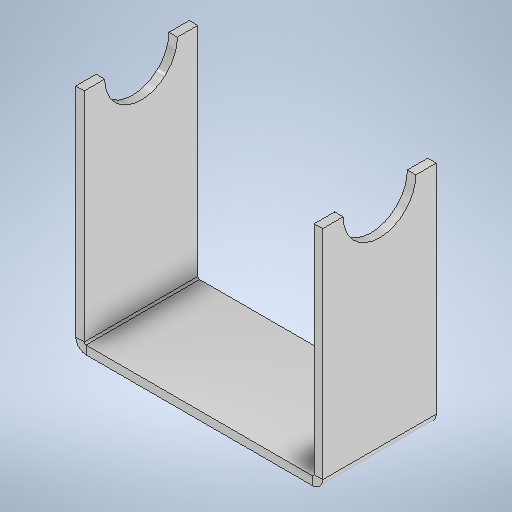
# Autodesk Inventor part: axis_10_top_frame
Saved by Autodesk Inventor 2025.2 (Build 292293000, 293)
## iProperties
Created: 2025-05-04
Part Number: axis_10_top_frame
Material: Aluminum 6061-AHC
Document SubType Name: Sheet Metal
Designer: User
Density: 2.7 g/cm^3
Sheet Metal Rule: Default_mm
Appearance: Aluminum - Dark
Author: User
Autodesk Inventor part; units mm, degrees
ref_plane "YZ Plane" through (0, 0, 0) normal (1, 0, 0) x (0, 1, 0)
ref_plane "XZ Plane" through (0, 0, 0) normal (0, 1, 0) x (-1, 0, 0)
ref_plane "XY Plane" through (0, 0, 0) normal (0, 0, 1) x (1, 0, 0)
sketch "Sketch1" plane through (0, 0, 0) normal (0, 1, 0) x (-1, 0, 0)
  line L0 (20.25, -10) -> (-20.25, -10)
  line L1 (-20.25, -10) -> (-20.25, 10)
  line L2 (-20.25, 10) -> (20.25, 10)
  line L3 (20.25, 10) -> (20.25, -10)
  point P0 (0, 0)
  dimension "d0" = 40.5
  dimension "d1" = 20
  dimension "d2" = 10
  dimension "d3" = 20.25
  measures "d0" distance of L0.start L0.end
  measures "d1" distance of L2.end L0.start
  measures "d2" distance from line of L0 point (0, 0)
  measures "d3" distance from line of point (0, 0) L3
extrude "Plate1" add sketch "Sketch1" along normal blind 1.5
sketch "Sketch2" plane through (21.75, 0, -10) normal (-1, 0, 0) x (0, -1, 0)
  line L0 (0, 20) -> (0, 0)
  line L1 (0, 0) -> (-50, 0)
  line L2 (-50, 0) -> (-50, 20)
  line L3 (-50, 20) -> (0, 20)
  constraints: 8 end point
edge flange "Flange1" height 50 angle 90 thickness 1.5 bend radius 0.31 thickness toward (-1, 0, 0) relief straight relief width 1.5 relief depth 0.75 edges at (20.25, 1.5, 0) wall of the first edge with corners at (21.75, 0, 10) (21.75, 0, -10) (21.75, 50, -10) (21.75, 50, 10)
bend "Bend1"
corner "Corner1"
sketch "Sketch3" plane through (-21.75, 0, 10) normal (1, 0, 0) x (0, 1, 0)
  line L0 (0, -20) -> (0, 0)
  line L1 (0, 0) -> (50, 0)
  line L2 (50, 0) -> (50, -20)
  line L3 (50, -20) -> (0, -20)
  constraints: 8 end point
edge flange "Flange2" height 50 angle 90 thickness 1.5 bend radius 0.31 thickness toward (1, 0, 0) relief straight relief width 1.5 relief depth 0.75 edges at (-20.25, 1.5, 0) wall of the first edge with corners at (-21.75, 0, -10) (-21.75, 0, 10) (-21.75, 50, 10) (-21.75, 50, -10)
bend "Bend2"
corner "Corner2"
sketch "Sketch4" plane through (21.75, 50, 10) normal (1, 0, 0) x (0, 0, -1)
  circle A0 centre (10, -9.9) radius 6.4
  line L0 (0, 0) -> (20, 0) projected
  line L1 (20, 0) -> (20, -48.19) projected
  point P0 (10, -50)
  dimension "d25" = 9.9
  dimension "d26" = 12.8
  dimension "d27" = 10
  constraints: 1 centre point
  measures "d25" distance from line of A0.centre L0
  measures "d26" diameter of A0
  measures "d27" distance from line of L1 A0.centre
extrude "Extrusion1" cut sketch "Sketch4" against normal blind 50
sketch "Sketch5" plane through (21.75, 50, 10) normal (1, 0, 0) x (0, 0, -1)
  circle A0 centre (10, -9.9) radius 6.4 projected
  line L0 (0, 0) -> (20, 0) projected
  line L1 (-4, 0) -> (24, 0)
  line L2 (24, 0) -> (24, -9.9)
  line L3 (24, -9.9) -> (-4, -9.9)
  line L4 (-4, -9.9) -> (-4, 0)
  line L5 (0, -48.19) -> (0, 0) projected
  point P0 (10, -50)
  dimension "d30" = 9.9
  dimension "d31" = 28
  dimension "d32" = 4
  constraints: 8 end point, 2 parallel, 1 horizontal, 1 perpendicular, 1 point on line
  measures "d30" distance of L3.end L1.start
  measures "d31" distance of L1.start L1.end
  measures "d32" distance between parallel lines of L5 L4
extrude "Extrusion2" cut sketch "Sketch5" against normal blind 50 contours L3 A0 | A0 L3 L5 L0 L1 L2 | L3 L4 L1 L5 picked at (9.2435, -7.9053)
equation "\"d4\" = Thickness"
equation "\"d5\" = BendReliefWidth"
equation "\"d6\" = BendReliefDepth"
equation "\"d7\" = MinimumRemnant"
equation "\"d8\" = TransitionRadius"
equation "\"d11\" = BendRadius"
equation "\"d12\" = CornerReliefSize"
equation "\"d13\" = GapSize"
equation "\"d14\" = JacobiRadiusSize"
equation "\"d15\" = BendReliefWidth"
equation "\"d16\" = BendReliefDepth"
equation "\"d17\" = MinimumRemnant"
equation "\"d18\" = TransitionRadius"
equation "\"d21\" = BendRadius"
equation "\"d22\" = CornerReliefSize"
equation "\"d23\" = GapSize"
equation "\"d24\" = JacobiRadiusSize"
equation "\"BendReliefWidth\" = Thickness"
equation "\"BendReliefDepth\" = 0.5 * Thickness"
equation "\"CornerReliefSize\" = 4 * Thickness"
equation "\"MinimumRemnant\" = 2 * Thickness"
equation "\"TransitionRadius\" = BendRadius"
equation "\"JacobiRadiusSize\" = BendRadius"
equation "\"GapSize\" = Thickness"
equation "\"Thickness\" = 1.5"
equation "\"BendRadius\" = 0.31"
body "Solid1"
